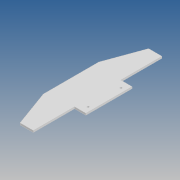
# Autodesk Inventor part: KB33-046-004-008 - Центральная правая боковая пластина
Saved by Autodesk Inventor 2020 (Build 240168000, 168)
## iProperties
Created: 2021-06-25
Part Number: KB33-046-004-008 - Центральная правая боковая пластина
Material: Типовые
Document SubType Name: Modeling
Designer: Петров Иван
Density: 1 g/cm^3
Appearance: По умолчанию
Mass: 70.1336 g
Surface Area: 379.707 cm^2
Volume: 70.1336 cm^3
Author: Петров Иван
Autodesk Inventor part; units mm, degrees
ref_plane "YZ Plane" through (0, 0, 0) normal (1, 0, 0) x (0, 1, 0)
ref_plane "XZ Plane" through (0, 0, 0) normal (0, 1, 0) x (-1, 0, 0)
ref_plane "XY Plane" through (0, 0, 0) normal (0, 0, 1) x (1, 0, 0)
sketch "Эскиз1" plane through (2.236, 0, -46.8876) normal (0, 1, 0) x (-1, 0, 0)
  line L0 (-10.528, 98.8876) -> (15, 98.8876)
  line L1 (15, 98.8876) -> (15, -5.1124)
  line L2 (15, -5.1124) -> (-10.528, -5.1124)
  line L3 (-10.528, -5.1124) -> (-10.528, 98.8876)
  point P0 (0, 0)
  dimension "d0" = 25.528
  dimension "d1" = 104
  constraints: 8 end point, 2 parallel, 1 horizontal, 1 perpendicular
  measures "d0" distance of L1.end L2.end
  measures "d1" distance of L0.end L1.end
extrude "Выдавливание1" add sketch "Эскиз1" along normal blind 4
sketch "Эскиз2" plane through (2.236, 4, -46.8876) normal (0, 1, 0) x (0, 0, -1)
  circle A0 centre (-9.8876, -0.528) radius 2 projected
  circle A1 centre (-83.8876, -0.528) radius 2 projected
  point P0 (0, 0)
extrude "Выдавливание2" cut sketch "Эскиз2" against normal blind 4
sketch "Эскиз3" plane through (2.236, 4, -46.8876) normal (0, 1, 0) x (1, 0, 0)
  line L0 (-45, -191.6906) -> (-15, -191.6906)
  line L1 (-15, -191.6906) -> (-15, 97.9154)
  line L2 (-15, 97.9154) -> (-45, 97.9154)
  line L3 (-45, 97.9154) -> (-45, -191.6906)
  line L4 (-15, -98.8876) -> (10.528, -98.8876) projected
  line L5 (10.528, 5.1124) -> (-15, 5.1124) projected
  point P0 (-2.236, -46.8876)
  dimension "d8" = 92.803
  dimension "d9" = 92.803
  dimension "d10" = 30
  constraints: 8 end point, 2 parallel, 1 horizontal, 1 perpendicular, 1 point on line
  measures "d8" distance between parallel lines of L4 L0
  measures "d9" distance between parallel lines of L2 L5
  measures "d10" distance between parallel lines of L1 L3
extrude "Выдавливание3" add sketch "Эскиз3" against normal blind 4
sketch "Эскиз4" plane through (2.236, 4, -46.8876) normal (0, 1, 0) x (1, 0, 0)
  line L0 (-45, -191.6906) -> (-45, 97.9154) projected
  line L1 (-45, -191.6906) -> (-75, -109.2663)
  line L2 (-75, -109.2663) -> (-75, 15.491)
  line L3 (-75, 15.491) -> (-45, 97.9154)
  line L4 (-2.236, -46.8876) -> (-20.0662, -46.8876)
  dimension "d13" = 30
  dimension "d14" = 20
  constraints: 8 end point, 1 horizontal, 1 parallel, 1 other
  measures "d13" distance between parallel lines of L0 L2
  measures "d14" angle of L0 L3
extrude "Выдавливание4" add sketch "Эскиз4" against normal blind 4
